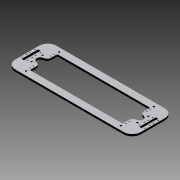
# Autodesk Inventor part: GANTRY BACK
Saved by Autodesk Inventor 2013 (Build 170138000, 138)
## iProperties
Created: 2014-06-16
Part Number: GANTRY BACK
Material: Generic
Document SubType Name: Modeling
Designer: employee
Density: 1 g/cm^3
Author: employee
Autodesk Inventor part; units mm, degrees
ref_plane "YZ Plane" through (0, 0, 0) normal (1, 0, 0) x (0, 1, 0)
ref_plane "XZ Plane" through (0, 0, 0) normal (0, 1, 0) x (-1, 0, 0)
ref_plane "XY Plane" through (0, 0, 0) normal (0, 0, 1) x (1, 0, 0)
sketch "Sketch1" plane through (0, 0, 0) normal (0, 0, 1) x (1, 0, 0)
  line L0 (0, 0) -> (-130, 0) construction
  line L1 (-130, 0) -> (-130, 70) construction
  line L2 (-130, 70) -> (0, 70) construction
  line L3 (0, 70) -> (0, 0) construction
  line L4 (-167.75, 0) -> (-167.75, 24)
  line L5 (-167.75, 24) -> (-175.25, 24)
  line L6 (-175.25, 24) -> (-175.25, 0)
  line L7 (-175.25, 0) -> (-183, 0)
  line L8 (-183, 0) -> (-183, 60)
  line L9 (-183, 60) -> (0, 60)
  line L10 (0, 60) -> (0, 40)
  line L11 (0, 40) -> (-135, 40)
  line L12 (-135, 40) -> (-135, 32)
  line L13 (-135, 32) -> (-145, 32)
  line L14 (-145, 32) -> (-145, 28)
  line L15 (-145, 28) -> (-135, 28)
  line L16 (-135, 28) -> (-135, 0)
  line L17 (-167.75, 0) -> (-135, 0)
  circle A0 centre (-138, 48) radius 8 construction
  circle A1 centre (-154, 16) radius 8 construction
  circle A2 centre (-154, 16) radius 2.5
  circle A3 centre (-138, 48) radius 2.5
  line L18 (-179, 24) -> (-164, 24) construction
  line L19 (-164, 24) -> (-164, 0) construction
  line L20 (-164, 0) -> (-179, 0) construction
  line L21 (-179, 0) -> (-179, 24) construction
  point P0 (-145, 30)
  point P1 (0, 50)
  point P2 (-171.5, 24)
  dimension "d0" = 130
  dimension "d1" = 70
  dimension "d2" = 30
  dimension "d3" = 20
  dimension "d4" = 4
  dimension "d5" = 10
  dimension "d6" = 10
  dimension "d7" = 145
  dimension "d8" = 16
  dimension "d9" = 16
  dimension "d10" = 16
  dimension "d11" = 7.5
  dimension "d13" = 24
  dimension "d14" = 11.5
  dimension "d15" = 183
  dimension "d18" = 5
  dimension "d29" = 15
  dimension "d31" = 10
  dimension "d38" = 18
  constraints: 44 end point, 12 parallel, 5 perpendicular, 4 centre point, 4 midpoint, 3 point on line, 2 coincident, 2 collinear, 2 equal radius, 2 horizontal, 1 horizontal alignment, 1 tangent, 1 vertical alignment
  measures "d0" distance of L0.start L0.end
  measures "d1" distance of L2.end L0.start
  measures "d2" distance from line of point (-145, 30) L17
  measures "d3" distance between parallel lines of L9 L11
  measures "d4" distance between parallel lines of L13 L15
  measures "d5" distance of L12.end L13.end
  measures "d6" distance from line of L11 point (-145, 30)
  measures "d7" horizontal distance of L0.start L14.end
  measures "d8" diameter of A0
  measures "d9" distance from line of A1.centre L17
  measures "d10" horizontal distance of A0.centre A1.centre
  measures "d11" distance between parallel lines of L4 L6
  measures "d13" distance from line of point (-171.5, 24) L7
  measures "d14" distance from line of point (-171.5, 24) L8
  measures "d15" distance of L0.start L7.end
  measures "d18" diameter of A2
  measures "d29" distance of L18.start L18.end
  measures "d31" distance from line of A1.centre L19
  measures "d38" vertical distance of A0.centre point (-145, 30)
extrude "Extrusion1" add sketch "Sketch1" along normal blind 5.715
fillet "Fillet1" radius 2 1 edges at (-135, 40, 2.8575)
fillet "Fillet1" radius 25 1 edges at (-183, 60, 2.8575)
sketch "Sketch2" plane through (0, 0, 5.715) normal (0, 0, 1) x (1, 0, 0)
  line L0 (-183, 0) -> (-175.25, 0) projected
  line L1 (-175.25, 0) -> (-175.25, 24) projected
  line L2 (-175.25, 24) -> (-167.75, 24) projected
  line L3 (-145, 28) -> (-145, 32) projected
  line L4 (-145, 32) -> (-135, 32) projected
  line L5 (-142, 34) -> (-138, 34)
  line L6 (-138, 34) -> (-138, 26) construction
  line L7 (-138, 26) -> (-142, 26)
  line L8 (-142, 26) -> (-142, 34) construction
  line L9 (-142, 26) -> (-138, 26)
  line L10 (-138, 26) -> (-138, 24.5)
  line L11 (-138, 24.5) -> (-142, 24.5)
  line L12 (-142, 24.5) -> (-142, 26)
  line L13 (-142, 34) -> (-138, 34)
  line L14 (-138, 34) -> (-138, 35.5)
  line L15 (-138, 35.5) -> (-142, 35.5)
  line L16 (-142, 35.5) -> (-142, 34)
  line L17 (-179, 21) -> (-164, 21) construction
  line L18 (-164, 21) -> (-164, 3) construction
  line L19 (-164, 3) -> (-179, 3) construction
  line L20 (-179, 3) -> (-179, 21) construction
  line L21 (-164, 3) -> (-162.5, 3)
  line L22 (-162.5, 3) -> (-162.5, 7)
  line L23 (-162.5, 7) -> (-164, 7)
  line L24 (-164, 7) -> (-164, 3)
  line L25 (-164, 21) -> (-162.5, 21)
  line L26 (-162.5, 21) -> (-162.5, 17)
  line L27 (-162.5, 17) -> (-164, 17)
  line L28 (-164, 17) -> (-164, 21)
  line L29 (-179, 21) -> (-180.5, 21)
  line L30 (-180.5, 21) -> (-180.5, 17)
  line L31 (-180.5, 17) -> (-179, 17)
  line L32 (-179, 17) -> (-179, 21)
  line L33 (-179, 3) -> (-180.5, 3)
  line L34 (-180.5, 3) -> (-180.5, 7)
  line L35 (-180.5, 7) -> (-179, 7)
  line L36 (-179, 7) -> (-179, 3)
  point P0 (0, 0)
  point P1 (-140, 34)
  point P2 (-140, 32)
  point P3 (-142, 30)
  point P4 (-145, 30)
  point P5 (-171.5, 21)
  point P6 (-171.5, 24)
  point P7 (-179, 12)
  point P8 (-175.25, 12)
  point P9 (-180.5, 5)
  dimension "d21" = 8
  dimension "d23" = 1.5
  dimension "d24" = 4
  dimension "d25" = 5
  dimension "d26" = 7.5
  constraints: 64 end point, 16 parallel, 9 equal length, 9 midpoint, 8 horizontal, 8 perpendicular, 2 horizontal alignment, 2 vertical alignment, 1 point on line
  measures "d21" distance of L5.end L6.end
  measures "d23" distance of L5.end L14.end
  measures "d24" distance of L14.end L15.end
  measures "d25" distance from line of point (-180.5, 5) L0
  measures "d26" horizontal distance of L19.end point (-171.5, 24)
extrude "Extrusion2" cut sketch "Sketch2" against normal through all
mirror "Mirror1" about plane through (-167.75, 0, 0) normal (0, -1, 0) of "Extrusion1", "Fillet1", "Extrusion2"
mirror "Mirror2" about plane through (0, -40, 0) normal (1, 0, 0) of "Extrusion1", "Fillet1", "Mirror1", "Extrusion2"
sketch "Sketch3" plane through (0, 0, 5.715) normal (0, 0, 1) x (1, 0, 0)
  line L0 (-167.75, 24) -> (-167.75, -24) projected
  line L1 (-135, 28) -> (-135, -28) projected
  line L2 (-145, 28) -> (-145, 32) projected
  arc A0 (-146.1724, 9.931) -> (-135, 22.5) centre (-147.6562, 22.5) ccw
  arc A1 (-146.1724, 9.931) -> (-146.1724, -9.931) centre (-145, 0) ccw
  arc A2 (-135, -22.5) -> (-146.1724, -9.931) centre (-147.6562, -22.5) ccw
  line L3 (-135, 0) -> (-155, 0)
  point P0 (0, 0)
  point P1 (-167.75, 0)
  point P2 (-145, 30)
  dimension "d32" = 7.5
  dimension "d34" = 20
  dimension "d35" = 10
  constraints: 7 point on circle, 4 tangent, 3 centre point, 3 midpoint, 2 end point, 2 point on line, 1 equal radius, 1 horizontal alignment
  measures "d32" vertical distance of A0.end point (-145, 30)
  measures "d34" distance of L3.start L3.end
  measures "d35" radius of A1
extrude "Extrusion3" cut sketch "Sketch3" against normal through all
mirror "Mirror3" about plane through (0, 0, 0) normal (1, 0, 0) of "Extrusion3"
sketch "Sketch5" plane through (0, 0, 5.715) normal (0, 0, 1) x (1, 0, 0)
  line L0 (135, -28) -> (145, -28) projected
  line L1 (145, -28) -> (145, -32) projected
  line L2 (145, -32) -> (135, -32) projected
  line L3 (-145, -32) -> (-135, -32) projected
  line L4 (-145, -28) -> (-145, -32) projected
  line L5 (-135, -28) -> (-145, -28) projected
  line L6 (-135, -22.5) -> (-135, -28) projected
  line L7 (-135, 28) -> (-145, 28) projected
  line L8 (-145, 28) -> (-145, 32) projected
  line L9 (-145, 32) -> (-135, 32) projected
  line L10 (145, 32) -> (135, 32) projected
  line L11 (145, 28) -> (145, 32) projected
  line L12 (135, 28) -> (145, 28) projected
  line L13 (-135, -32) -> (-135, -28)
  line L14 (-135, 28) -> (-135, 32)
  line L15 (135, -32) -> (135, -28)
  line L16 (135, 32) -> (135, 28)
  point P0 (0, 0)
  constraints: 8 end point, 3 collinear, 1 parallel
extrude "Extrusion4" add sketch "Sketch5" against normal up to surface (5.715 mm away)
body "Solid1"
